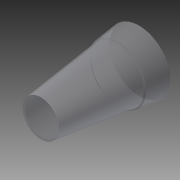
# Autodesk Inventor part: PopcornCup
Saved by Autodesk Inventor 2014 SP1 (Build 180222100, 222)
## iProperties
Created: 2015-04-12
Part Number: PopcornCup
Material: Polycarbonate, Clear
Document SubType Name: Modeling
Designer: david
Density: 1.2 g/cm^3
Appearance: Polycarbonate - Clear
Mass: 95.5435 g
Surface Area: 802.446 cm^2
Volume: 79.6195 cm^3
Author: david
Autodesk Inventor part; units mm, degrees
ref_plane "YZ Plane" through (0, 0, 0) normal (1, 0, 0) x (0, 1, 0)
ref_plane "XZ Plane" through (0, 0, 0) normal (0, 1, 0) x (-1, 0, 0)
ref_plane "XY Plane" through (0, 0, 0) normal (0, 0, 1) x (1, 0, 0)
sketch "Sketch1" plane through (0, 0, 0) normal (0, 0, 1) x (1, 0, 0)
  line L0 (0, 0) -> (29, 0)
  line L1 (29, 0) -> (43.462, 119.715)
  line L2 (43.462, 119.715) -> (45.3715, 121.8246)
  line L3 (45.3715, 121.8246) -> (49.5, 156)
  line L4 (49.5, 156) -> (0, 156) construction
  line L5 (0, 156) -> (0, 0) construction
  line L6 (-56.2795, 168.8188) -> (80.6142, 168.8188) construction
  line L7 (80.6142, 168.8188) -> (80.6142, -29.1812) construction
  line L8 (80.6142, -29.1812) -> (-56.2795, -29.1812) construction
  line L9 (-56.2795, -29.1812) -> (-56.2795, 168.8188) construction
  line L10 (0, 0) -> (0, 2)
  line L11 (0, 2) -> (27.2271, 2)
  line L12 (27.2271, 2) -> (41.5527, 120.5859)
  line L13 (41.5527, 120.5859) -> (43.4622, 122.6955)
  line L14 (43.4622, 122.6955) -> (47.4855, 156)
  line L15 (49.5, 156) -> (47.4855, 156)
  dimension "d1" = 29
  dimension "d2" = 49.5
  dimension "d3" = 156
  dimension "d13" = 198
  dimension "d24" = 2
  dimension "d25" = 2
  dimension "d26" = 2
  dimension "d27" = 2
  constraints: 24 end point, 5 parallel, 2 perpendicular, 2 point on line, 1 collinear, 1 horizontal, 2 other
  measures "d1" distance of L0.start L0.end
  measures "d2" distance of L3.end L4.end
  measures "d3" distance of L4.end L0.start
  measures "d13" distance of L6.end L7.end
  measures "d24" distance between parallel lines of L0 L11
  measures "d25" distance between parallel lines of L1 L12
  measures "d26" distance between parallel lines of L2 L13
  measures "d27" distance between parallel lines of L3 L14
revolve "Revolution1" add sketch "Sketch1" angle 360 about axis through (0, 156, 0) along (0, -1, 0)
equation "\"d24\" = PopcornCup_Thickness"
equation "\"d25\" = PopcornCup_Thickness"
equation "\"d26\" = PopcornCup_Thickness"
equation "\"d27\" = PopcornCup_Thickness"
equation "\"PopcornCup_Thickness\" = 2"
equation "\"PopcornCup_Base_DiameterMax\" = 58"
body "Solid1"
